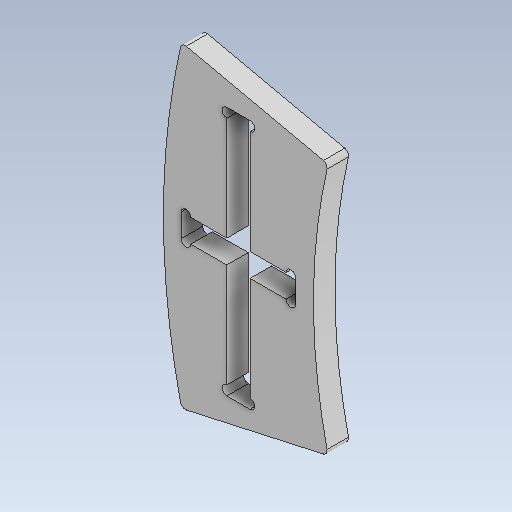
# Autodesk Inventor part: Feet
Saved by Autodesk Inventor 2020 (Build 240168000, 168)
## iProperties
Created: 2020-03-12
Part Number: Feet
Material: Generic
Document SubType Name: Modeling
Designer: Daniel Wikman
Density: 1 g/cm^3
Appearance: Default
Author: Daniel Wikman
Autodesk Inventor part; units mm, degrees
ref_plane "YZ Plane" through (0, 0, 0) normal (1, 0, 0) x (0, 1, 0)
ref_plane "XZ Plane" through (0, 0, 0) normal (0, 1, 0) x (-1, 0, 0)
ref_plane "XY Plane" through (0, 0, 0) normal (0, 0, 1) x (1, 0, 0)
sketch "Sketch1" plane through (0, 0, 0) normal (0, 0, 1) x (1, 0, 0)
  line L0 (-3.25, 35) -> (3.25, 35)
  arc A0 (-13.3333, 3.25) -> (-16, 3.25) centre (-14.6667, 3.25) ccw
  arc A1 (16.0137, 3.25) -> (13.347, 3.25) centre (14.6803, 3.25) ccw
  arc A2 (-3.25, 35) -> (-3.25, 32.3333) centre (-3.25, 33.6667) ccw
  arc A3 (3.25, 32.3333) -> (3.25, 35) centre (3.25, 33.6667) ccw
  line L1 (3.25, 32.3333) -> (3.25, 3.25)
  line L2 (-3.25, 3.25) -> (-3.25, 32.3333)
  line L3 (13.347, 3.25) -> (3.25, 3.25)
  line L4 (-3.25, 3.25) -> (-13.3333, 3.25)
  line L5 (-15.9119, 44.3695) -> (25.0953, 35.2784)
  line L6 (-15.9119, -44.3695) -> (25.0953, -35.2784)
  line L7 (107.2341, 51.0746) -> (107.2341, -58.8764)
  arc A4 (-15.9119, 44.3695) -> (-15.9119, -44.3695) centre (175, 0) ccw
  arc A5 (25.0953, 35.2784) -> (25.0953, -35.2784) centre (175, 0) ccw
  line L8 (-24.8255, 0) -> (30.5939, 0)
  line L9 (-16, 3.25) -> (-16, 0)
  line L10 (16.0137, 3.25) -> (16.0137, 0)
  line L11 (-3.25, -35) -> (3.25, -35)
  arc A6 (-16, -3.25) -> (-13.3333, -3.25) centre (-14.6667, -3.25) ccw
  arc A7 (13.347, -3.25) -> (16.0137, -3.25) centre (14.6803, -3.25) ccw
  arc A8 (-3.25, -32.3333) -> (-3.25, -35) centre (-3.25, -33.6667) ccw
  arc A9 (3.25, -35) -> (3.25, -32.3333) centre (3.25, -33.6667) ccw
  line L12 (3.25, -32.3333) -> (3.25, -3.25)
  line L13 (-3.25, -3.25) -> (-3.25, -32.3333)
  line L14 (13.347, -3.25) -> (3.25, -3.25)
  line L15 (-3.25, -3.25) -> (-13.3333, -3.25)
  line L16 (-16, -3.25) -> (-16, 0)
  line L17 (16.0137, -3.25) -> (16.0137, 0)
  point P0 (0, 0)
  dimension "d3" = 1.3333
  dimension "d4" = 2.6667
  dimension "d14" = 2.6667
  dimension "d15" = 1.3333
  dimension "d26" = 392
  dimension "d30" = 5
  dimension "d38" = 0
  dimension "d40" = 10.097
  dimension "d41" = 0
  dimension "d42" = 3.25
  dimension "d43" = 0
  constraints: 36 end point, 20 point on circle, 14 symmetric about line, 10 centre point, 3 horizontal, 2 perpendicular, 2 point on line, 1 coincident, 1 collinear, 1 parallel, 1 vertical, 4 other
  measures "d3" radius of A0
  measures "d4" diameter of A1
  measures "d14" diameter of A2
  measures "d15" radius of A3
  measures "d26" diameter of A4
  measures "d30" distance from line of L5 L0.end
  measures "d38" distance from line of A0.centre L4
  measures "d40" distance of L3.start L1.end
  measures "d41" distance from line of L3 A1.centre
  measures "d42" distance between parallel lines of L8 L4
  measures "d43" distance from line of point (0, 0) L8
extrude "Extrusion1" add sketch "Sketch1" along normal blind 6 contours A2 L2 L4 A0 L9 L8 A4 L5 A5 L10 A1 L3 L1 A3 L0 | L16 A6 L15 L13 A8 L11 A9 L12 L14 A7 L17 L8 A5 L6 A4
fillet "Fillet1" radius 1.3333 4 edges at (-15.9119, -44.3695, 3) (25.0953, -35.2784, 3) (25.0953, 35.2784, 3) (-15.9119, 44.3695, 3)
body "Solid1"
